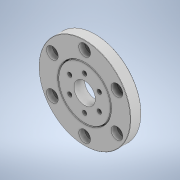
# Autodesk Inventor part: CRBTF105AT
Saved by Autodesk Inventor 2020.4 (Build 244396000, 396)
## iProperties
Created: 2021-09-21
Part Number: CRBTF105AT
Material: 一般
Document SubType Name: Modeling
Designer: Masato
Density: 1 g/cm^3
Appearance: 既定
Author: Masato
Autodesk Inventor part; units mm, degrees
ref_plane "YZ Plane" through (0, 0, 0) normal (1, 0, 0) x (0, 1, 0)
ref_plane "XZ Plane" through (0, 0, 0) normal (0, 1, 0) x (-1, 0, 0)
ref_plane "XY Plane" through (0, 0, 0) normal (0, 0, 1) x (1, 0, 0)
sketch "スケッチ1" plane through (0, 0, 0) normal (0, 0, 1) x (1, 0, 0)
  circle A0 centre (0, 0) radius 21.5
  circle A1 centre (0, 0) radius 5
  circle A2 centre (0, 0) radius 12.6
  circle A3 centre (0, 0) radius 12.1
  line L0 (0, 21.5) -> (0, 0) construction
  circle A4 centre (0, 17.5) radius 2.75
  circle A5 centre (-15.1554, 8.75) radius 2.75
  circle A6 centre (-15.1554, -8.75) radius 2.75
  circle A7 centre (0, -17.5) radius 2.75
  circle A8 centre (15.1554, -8.75) radius 2.75
  circle A9 centre (15.1554, 8.75) radius 2.75
  point P0 (0, 8)
  point P1 (-6.9282, 4)
  point P2 (-6.9282, -4)
  point P3 (0, -8)
  point P4 (6.9282, -4)
  point P5 (6.9282, 4)
  dimension "d0" = 43
  dimension "d1" = 10
  dimension "d2" = 25.2
  dimension "d3" = 24.2
  dimension "d4" = 8
  dimension "d5" = 17.5
  dimension "d10" = 5.5
  dimension "d13" = 360
  constraints: 10 coincident, 9 centre point, 2 end point, 2 point on line, 1 vertical, 1 vertical alignment, 27 other
  measures "d1" diameter of A1
  measures "d2" diameter of A2
  measures "d3" diameter of A3
  measures "d4" distance of point (0, 0) point (0, 8)
  measures "d5" distance of point (0, 0) point (0, 17.5)
  measures "d10" diameter of A4
extrude "押し出し1" add sketch "スケッチ1" along normal blind 5
extrude "押し出し2" add sketch "スケッチ1" along normal blind 2.2 contours A4 | A5 | A6 | A7 | A8 | A9
hole "穴1" at (0, 17.5, 0) at (15.1554, 8.75, 0) at (15.1554, -8.75, 0) at (0, -17.5, 0) at (-15.1554, -8.75, 0) at (-15.1554, 8.75, 0) direction (0, 0, 1) diameter 2.9 end through all
hole "穴2" at (0, 8, 0) at (-6.9282, 4, 0) at (-6.9282, -4, 0) at (0, -8, 0) at (6.9282, -4, 0) at (6.9282, 4, 0) direction (0, 0, 1) diameter 2.013 end through all thread size "M2.5x0.45" class "6H" standard "ISO Metric profile"
fillet "フィレット1" radius 0.15 2 edges at (-21.5, 0, 5) (-21.5, 0, 0)
